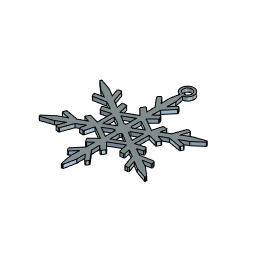
Snowflake 3 (Autodesk Fusion 360 design; units mm, degrees)
Autodesk Fusion 360 part; units mm, degrees
note: some values were not read from the file. Chosen so that the rebuilt part matches the saved one: which bodies a step acts on.
sketch "Sketch1" plane through (0, 0, 0) normal (0, 0, 1) x (1, 0, 0)
  line L0 (4.1638, 67.6877) -> (3.0782, 8.4572)
  line L1 (3.0782, 8.4572) -> (0, 0)
  line L2 (0, 0) -> (-3.0782, 8.4572)
  line L3 (-3.0782, 8.4572) -> (-4.1638, 67.6877)
  line L4 (-4.1638, 67.6877) -> (-1.1108, 83.3937)
  line L5 (-0.62, 83.7983) -> (0.62, 83.7983)
  line L6 (1.1108, 83.3937) -> (4.1638, 67.6877)
  line L7 (0, 0) -> (0, 83.7983) construction
  arc A0 (-0.62, 83.7983) -> (-1.1108, 83.3937) centre (-0.62, 83.2983) ccw
  arc A1 (1.1108, 83.3937) -> (0.62, 83.7983) centre (0.62, 83.2983) ccw
  dimension "d355" = 40
  dimension "d356" = 0.5
  dimension "d357" = 0.5
  dimension "d358" = 9
  dimension "d359" = 2.1
  dimension "d360" = 22
  dimension "d361" = 16
  dimension "d362" = 1.24
  constraint coincident L1.end L2.start
  constraint horizontal L5
  constraint vertical L7
  constraint symmetric L4 L6 L7
  constraint symmetric L0 L3 L7
  constraint symmetric L1 L2 L7
  constraint coincident L5 L7.end
  constraint tangent L4 A0
  constraint tangent L5 A0
  constraint tangent L5 A1
  constraint tangent L6 A1
  measures "d355" angle of L1 L2
  measures "d356" radius of A0
  measures "d357" radius of A1
  measures "d358" distance of L0.end L1.end
  measures "d359" angle of L0 L3
  measures "d360" angle of L4 L6
  measures "d361" distance of L0.start L6.start
  measures "d362" distance of L5.start L5.end
extrude "Extrude1" add sketch "Sketch1" along normal blind 5 makes body 1
pattern_circular "C-Pattern1" count 6 over 360 about axis through (0, 0, 1.75) along (0, 0, 1) of bodies 1 makes body 2 at (-42.0339, 23.0835, 0) makes body 3 at (-41.0079, -24.8607, 0) makes body 4 at (1.0261, -47.9442, 0) makes body 5 at (42.0339, -23.0835, 0) makes body 6 at (41.0079, 24.8607, 0)
sketch "Sketch2" plane through (0, 0, 0) normal (0, 0, 1) x (1, 0, 0)
  line L0 (1.1108, 83.3937) -> (4.1638, 67.6877)
  line L1 (4.1638, 67.6877) -> (3.0782, 8.4572)
  line L2 (3.0782, 8.4572) -> (0, 0)
  line L3 (0, 0) -> (-3.0782, 8.4572)
  line L4 (-3.0782, 8.4572) -> (-4.1638, 67.6877)
  line L5 (-4.1638, 67.6877) -> (-1.1108, 83.3937)
  arc A0 (-0.62, 83.7983) -> (-1.1108, 83.3937) centre (-0.62, 83.2983) ccw
  line L6 (-0.62, 83.7983) -> (0.62, 83.7983)
  arc A1 (1.1108, 83.3937) -> (0.62, 83.7983) centre (0.62, 83.2983) ccw
  line L7 (72.7765, 40.7349) -> (60.7011, 30.2379)
  line L8 (60.7011, 30.2379) -> (8.8633, 1.5628)
  line L9 (8.8633, 1.5628) -> (0, 0)
  line L10 (0, 0) -> (5.7851, 6.8944)
  line L11 (5.7851, 6.8944) -> (56.5374, 37.4498)
  line L12 (56.5374, 37.4498) -> (71.6657, 42.6589)
  arc A2 (72.2615, 42.4361) -> (71.6657, 42.6589) centre (71.8285, 42.1861) ccw
  line L13 (72.2615, 42.4361) -> (72.8815, 41.3622)
  arc A3 (72.7765, 40.7349) -> (72.8815, 41.3622) centre (72.4485, 41.1122) ccw
  line L14 (3.0782, 8.4572) -> (3.9851, 6.9024)
  line L15 (3.9851, 6.9024) -> (5.7851, 6.8944)
  line L16 (3.9851, 6.9024) -> (0, 0) construction
  dimension "d367" = 1.8
  constraint coincident L1.end L2.start
  constraint coincident L10.end L11.start
  constraint coincident L2.end L3.start
  constraint symmetric L2 L10 L16
  measures "d367" distance of L1.end L14.end
extrude "Extrude2" add sketch "Sketch2" along normal up to surface (5 mm away) separate body contours L2 L10 L14 L15 makes body 7
pattern_circular "C-Pattern2" count 6 over 360 about axis through (0, 0, 1.75) along (0, 0, 1) of bodies 7 makes body 8 at (-1.0261, 2.8191, 1.6667) makes body 9 at (-2.9544, 0.5209, 1.6667) makes body 10 at (-1.9284, -2.2981, 1.6667) makes body 11 at (1.0261, -2.8191, 1.6667) makes body 12 at (2.9544, -0.5209, 1.6667)
combine "Combine1" operation add target body 1 tool bodies 7 6 12 5 11 4 10 3 9 8 2
sketch "Sketch3" plane through (0, 0, 0) normal (0, 0, 1) x (1, 0, 0)
  line L0 (3.9453, 55.7691) -> (10.9697, 63.7874)
  line L1 (12.5222, 63.7282) -> (14.4807, 61.1147)
  line L2 (14.444, 59.8693) -> (3.7895, 47.2704)
  line L3 (3.7895, 47.2704) -> (3.9453, 55.7691)
  line L4 (-3.9453, 55.7691) -> (-10.9697, 63.7874)
  line L5 (-12.5222, 63.7282) -> (-14.4807, 61.1147)
  line L6 (-14.444, 59.8693) -> (-3.7895, 47.2704)
  line L7 (-3.7895, 47.2704) -> (-3.9453, 55.7691)
  line L8 (3.5792, 35.7959) -> (9.2878, 40.9035)
  line L9 (10.8187, 40.6617) -> (13.094, 36.7562)
  line L10 (12.9224, 35.5313) -> (3.407, 26.4)
  line L11 (3.407, 26.4) -> (3.5792, 35.7959)
  line L12 (-3.5792, 35.7959) -> (-9.2878, 40.9035)
  line L13 (-10.8187, 40.6617) -> (-13.094, 36.7562)
  line L14 (-12.9224, 35.5313) -> (-3.407, 26.4)
  line L15 (-3.407, 26.4) -> (-3.5792, 35.7959)
  line L16 (1.1108, 83.3937) -> (4.1638, 67.6877)
  line L17 (4.1638, 67.6877) -> (3.0782, 8.4572)
  line L18 (3.0782, 8.4572) -> (3.9851, 6.9024)
  line L19 (3.9851, 6.9024) -> (5.7851, 6.8944)
  line L20 (5.7851, 6.8944) -> (56.5374, 37.4498)
  line L21 (56.5374, 37.4498) -> (71.6657, 42.6589)
  arc A0 (72.2615, 42.4361) -> (71.6657, 42.6589) centre (71.8285, 42.1861) ccw
  line L22 (72.2615, 42.4361) -> (72.8815, 41.3622)
  arc A1 (72.7765, 40.7349) -> (72.8815, 41.3622) centre (72.4485, 41.1122) ccw
  line L23 (72.7765, 40.7349) -> (60.7011, 30.2379)
  line L24 (60.7011, 30.2379) -> (8.8633, 1.5628)
  line L25 (8.8633, 1.5628) -> (7.9702, 0)
  line L26 (7.9702, 0) -> (8.8633, -1.5628)
  line L27 (8.8633, -1.5628) -> (60.7011, -30.2379)
  line L28 (60.7011, -30.2379) -> (72.7765, -40.7349)
  arc A2 (72.8815, -41.3622) -> (72.7765, -40.7349) centre (72.4485, -41.1122) ccw
  line L29 (72.8815, -41.3622) -> (72.2615, -42.4361)
  arc A3 (71.6657, -42.6589) -> (72.2615, -42.4361) centre (71.8285, -42.1861) ccw
  line L30 (71.6657, -42.6589) -> (56.5374, -37.4498)
  line L31 (56.5374, -37.4498) -> (5.7851, -6.8944)
  line L32 (5.7851, -6.8944) -> (3.9851, -6.9024)
  line L33 (3.9851, -6.9024) -> (3.0782, -8.4572)
  line L34 (3.0782, -8.4572) -> (4.1638, -67.6877)
  line L35 (4.1638, -67.6877) -> (1.1108, -83.3937)
  arc A4 (0.62, -83.7983) -> (1.1108, -83.3937) centre (0.62, -83.2983) ccw
  line L36 (0.62, -83.7983) -> (-0.62, -83.7983)
  arc A5 (-1.1108, -83.3937) -> (-0.62, -83.7983) centre (-0.62, -83.2983) ccw
  line L37 (-1.1108, -83.3937) -> (-4.1638, -67.6877)
  line L38 (-4.1638, -67.6877) -> (-3.0782, -8.4572)
  line L39 (-3.0782, -8.4572) -> (-3.9851, -6.9024)
  line L40 (-3.9851, -6.9024) -> (-5.7851, -6.8944)
  line L41 (-5.7851, -6.8944) -> (-56.5374, -37.4498)
  line L42 (-56.5374, -37.4498) -> (-71.6657, -42.6589)
  arc A6 (-72.2615, -42.4361) -> (-71.6657, -42.6589) centre (-71.8285, -42.1861) ccw
  line L43 (-72.2615, -42.4361) -> (-72.8815, -41.3622)
  arc A7 (-72.7765, -40.7349) -> (-72.8815, -41.3622) centre (-72.4485, -41.1122) ccw
  line L44 (-72.7765, -40.7349) -> (-60.7011, -30.2379)
  line L45 (-60.7011, -30.2379) -> (-8.8633, -1.5628)
  line L46 (-8.8633, -1.5628) -> (-7.9702, 0)
  line L47 (-7.9702, 0) -> (-8.8633, 1.5628)
  line L48 (-8.8633, 1.5628) -> (-60.7011, 30.2379)
  line L49 (-60.7011, 30.2379) -> (-72.7765, 40.7349)
  arc A8 (-72.8815, 41.3622) -> (-72.7765, 40.7349) centre (-72.4485, 41.1122) ccw
  line L50 (-72.8815, 41.3622) -> (-72.2615, 42.4361)
  arc A9 (-71.6657, 42.6589) -> (-72.2615, 42.4361) centre (-71.8285, 42.1861) ccw
  line L51 (-71.6657, 42.6589) -> (-56.5374, 37.4498)
  line L52 (-56.5374, 37.4498) -> (-5.7851, 6.8944)
  line L53 (-5.7851, 6.8944) -> (-3.9851, 6.9024)
  line L54 (-3.9851, 6.9024) -> (-3.0782, 8.4572)
  line L55 (-3.0782, 8.4572) -> (-4.1638, 67.6877)
  line L56 (-4.1638, 67.6877) -> (-1.1108, 83.3937)
  arc A10 (-0.62, 83.7983) -> (-1.1108, 83.3937) centre (-0.62, 83.2983) ccw
  line L57 (-0.62, 83.7983) -> (0.62, 83.7983)
  arc A11 (1.1108, 83.3937) -> (0.62, 83.7983) centre (0.62, 83.2983) ccw
  line L58 (0, 83.7983) -> (0, 0) construction
  arc A12 (12.5222, 63.7282) -> (10.9697, 63.7874) centre (11.7219, 63.1285) ccw
  arc A13 (14.444, 59.8693) -> (14.4807, 61.1147) centre (13.6804, 60.515) ccw
  arc A14 (-10.9697, 63.7874) -> (-12.5222, 63.7282) centre (-11.7219, 63.1285) ccw
  arc A15 (-14.4807, 61.1147) -> (-14.444, 59.8693) centre (-13.6804, 60.515) ccw
  arc A16 (-9.2878, 40.9035) -> (-10.8187, 40.6617) centre (-9.9546, 40.1583) ccw
  arc A17 (-13.094, 36.7562) -> (-12.9224, 35.5313) centre (-12.23, 36.2528) ccw
  arc A18 (10.8187, 40.6617) -> (9.2878, 40.9035) centre (9.9546, 40.1583) ccw
  arc A19 (12.9224, 35.5313) -> (13.094, 36.7562) centre (12.23, 36.2528) ccw
  dimension "d372" = 1
  dimension "d373" = 1
  dimension "d374" = 1
  dimension "d375" = 10.66
  dimension "d376" = 3.2659
  dimension "d377" = 16.5
  dimension "d378" = 38.8131
  dimension "d379" = 40.17
  dimension "d380" = 1
  dimension "d381" = 1
  dimension "d382" = 2
  dimension "d383" = 4.52
  dimension "d384" = 7.66
  dimension "d385" = 47.13
  dimension "d386" = 26.4
  constraint collinear L11 L17
  constraint collinear L15 L55
  constraint collinear L7 L55
  constraint collinear L3 L17
  constraint midpoint L57 L58.start
  constraint coincident L58.end origin
  constraint symmetric L0 L4 L58
  constraint tangent L0 A12
  constraint tangent L1 A12
  constraint tangent L1 A13
  constraint tangent L2 A13
  constraint equal A12 A13
  constraint coincident L0.start L17
  constraint tangent L5 A14
  constraint tangent L4 A14
  constraint tangent L5 A15
  constraint tangent L6 A15
  constraint symmetric L1 L5 L58
  constraint symmetric L2 L6 L58
  constraint coincident L8.start L17
  constraint coincident L12.start L55
  constraint tangent L13 A16
  constraint tangent L12 A16
  constraint tangent L13 A17
  constraint tangent L14 A17
  constraint equal A16 A17
  constraint tangent L8 A18
  constraint tangent L9 A18
  constraint equal A16 A18
  constraint tangent L9 A19
  constraint tangent L10 A19
  constraint equal A16 A19
  constraint symmetric L8 L12 L58
  constraint symmetric L9 L13 L58
  constraint symmetric L10 L14 L58
  measures "d372" radius of A12
  measures "d373" radius of A14
  measures "d374" radius of A15
  measures "d375" distance of L0.start L0.end
  measures "d376" distance of L1.start L1.end
  measures "d377" distance of L2.end L2.start
  measures "d378" vertical distance of L2.end L17.end
  measures "d379" angle of L0 L17
  measures "d380" angle of L0 L2
  measures "d381" radius of A16
  measures "d382" angle of L8 L10
  measures "d383" distance of L9.start L9.end
  measures "d384" distance of L8.start L8.end
  measures "d385" angle of L8 L17
  measures "d386" vertical distance of L58.end L10.end
extrude "Extrude3" add sketch "Sketch3" along normal up to surface (5 mm away) separate body contours L0 L1 L2 L3 L17 A12 A13 | L8 L9 L10 L11 L17 A18 A19 | L4 L5 L6 L7 L55 A14 A15 | L12 L13 L14 L15 L55 A16 A17 makes body 13 at (6.6362, 32.5757, 0) makes body 14 at (-6.6362, 32.5757, 0) makes body 15 at (10.8925, 55.6697, 1.6667) makes body 16 at (-10.8925, 55.6697, 1.6667)
pattern_circular "C-Pattern3" count 6 over 360 about axis through (0, 0, 1.75) along (0, 0, 1) of bodies 13 14 15 16 makes body 17 at (-24.8933, 22.035, 0) makes body 18 at (-31.5295, -10.5407, 0) makes body 19 at (-6.6362, -32.5757, 0) makes body 20 at (24.8933, -22.035, 0) makes body 21 at (31.5295, 10.5407, 0) makes body 22 at (-31.5295, 10.5407, 0) makes body 23 at (-24.8933, -22.035, 0) makes body 24 at (6.6362, -32.5757, 0) makes body 25 at (31.5295, -10.5407, 0) makes body 26 at (24.8933, 22.035, 0) makes body 27 at (-42.7651, 37.268, 1.6667) makes body 28 at (-53.6576, -18.4016, 1.6667) makes body 29 at (-10.8925, -55.6697, 1.6667) makes body 30 at (42.7651, -37.268, 1.6667) makes body 31 at (53.6576, 18.4016, 1.6667) makes body 32 at (-53.6576, 18.4016, 3.3333) makes body 33 at (-42.7651, -37.268, 1.6667) makes body 34 at (10.8925, -55.6697, 3.3333) makes body 35 at (53.6576, -18.4016, 1.6667) makes body 36 at (42.7651, 37.268, 1.6667)
combine "Combine2" operation add target body 1 tool bodies 15 16 14 13 36 26 31 21 25 20 23 18 22 32 27 17 28 33 19 24 34 29 30 35
sketch "Sketch4" plane through (0, 0, 0) normal (0, 0, 1) x (1, 0, 0)
  line L0 (4.1458, 27.109) -> (21.4042, 17.1449)
  line L1 (3.3114, 21.1822) -> (16.6886, 13.4588)
  line L2 (1.1108, 83.3937) -> (4.1638, 67.6877)
  line L3 (4.1638, 67.6877) -> (3.9453, 55.7691)
  line L4 (3.9453, 55.7691) -> (10.9697, 63.7874)
  arc A0 (12.5222, 63.7282) -> (10.9697, 63.7874) centre (11.7219, 63.1285) ccw
  line L5 (12.5222, 63.7282) -> (14.4807, 61.1147)
  arc A1 (14.444, 59.8693) -> (14.4807, 61.1147) centre (13.6804, 60.515) ccw
  line L6 (14.444, 59.8693) -> (3.7895, 47.2704)
  line L7 (3.7895, 47.2704) -> (3.5792, 35.7959)
  line L8 (3.5792, 35.7959) -> (9.2878, 40.9035)
  arc A2 (10.8187, 40.6617) -> (9.2878, 40.9035) centre (9.9546, 40.1583) ccw
  line L9 (10.8187, 40.6617) -> (13.094, 36.7562)
  arc A3 (12.9224, 35.5313) -> (13.094, 36.7562) centre (12.23, 36.2528) ccw
  line L10 (12.9224, 35.5313) -> (3.407, 26.4)
  line L11 (3.407, 26.4) -> (3.0782, 8.4572)
  line L12 (3.0782, 8.4572) -> (3.9851, 6.9024)
  line L13 (3.9851, 6.9024) -> (5.7851, 6.8944)
  line L14 (5.7851, 6.8944) -> (21.1596, 16.1506)
  line L15 (21.1596, 16.1506) -> (24.3098, 28.9567)
  arc A4 (25.2848, 29.7179) -> (24.3098, 28.9567) centre (25.2808, 28.7179) ccw
  line L16 (25.2848, 29.7179) -> (29.8047, 29.7001)
  arc A5 (30.7796, 28.4952) -> (29.8047, 29.7001) centre (29.8008, 28.7001) ccw
  line L17 (30.7796, 28.4952) -> (29.2105, 20.9977)
  line L18 (29.2105, 20.9977) -> (39.0426, 26.917)
  line L19 (39.0426, 26.917) -> (44.6263, 42.4435)
  arc A6 (45.6866, 43.098) -> (44.6263, 42.4435) centre (45.5673, 42.1051) ccw
  line L20 (45.6866, 43.098) -> (48.9291, 42.7086)
  arc A7 (49.7567, 41.3938) -> (48.9291, 42.7086) centre (48.8099, 41.7157) ccw
  line L21 (49.7567, 41.3938) -> (46.3248, 31.3013)
  line L22 (46.3248, 31.3013) -> (56.5374, 37.4498)
  line L23 (56.5374, 37.4498) -> (71.6657, 42.6589)
  arc A8 (72.2615, 42.4361) -> (71.6657, 42.6589) centre (71.8285, 42.1861) ccw
  line L24 (72.2615, 42.4361) -> (72.8815, 41.3622)
  arc A9 (72.7765, 40.7349) -> (72.8815, 41.3622) centre (72.4485, 41.1122) ccw
  line L25 (72.7765, 40.7349) -> (60.7011, 30.2379)
  line L26 (60.7011, 30.2379) -> (50.2701, 24.4678)
  line L27 (50.2701, 24.4678) -> (60.7264, 22.3936)
  arc A10 (61.4513, 21.0196) -> (60.7264, 22.3936) centre (60.5318, 21.4128) ccw
  line L28 (61.4513, 21.0196) -> (60.1672, 18.0167)
  arc A11 (59.0703, 17.4258) -> (60.1672, 18.0167) centre (59.2478, 18.4099) ccw
  line L29 (59.0703, 17.4258) -> (42.8321, 20.3533)
  line L30 (42.8321, 20.3533) -> (32.7898, 14.7982)
  line L31 (32.7898, 14.7982) -> (40.0674, 12.4083)
  arc A12 (40.6234, 10.9616) -> (40.0674, 12.4083) centre (39.7554, 11.4582) ccw
  line L32 (40.6234, 10.9616) -> (38.3788, 7.0383)
  arc A13 (37.2322, 6.5745) -> (38.3788, 7.0383) centre (37.5108, 7.5349) ccw
  line L33 (37.2322, 6.5745) -> (24.5666, 10.2494)
  line L34 (24.5666, 10.2494) -> (8.8633, 1.5628)
  line L35 (8.8633, 1.5628) -> (7.9702, 0)
  line L36 (7.9702, 0) -> (8.8633, -1.5628)
  line L37 (8.8633, -1.5628) -> (24.5666, -10.2494)
  line L38 (24.5666, -10.2494) -> (37.2322, -6.5745)
  arc A14 (38.3788, -7.0383) -> (37.2322, -6.5745) centre (37.5108, -7.5349) ccw
  line L39 (38.3788, -7.0383) -> (40.6234, -10.9616)
  arc A15 (40.0674, -12.4083) -> (40.6234, -10.9616) centre (39.7554, -11.4582) ccw
  line L40 (40.0674, -12.4083) -> (32.7898, -14.7982)
  line L41 (32.7898, -14.7982) -> (42.8321, -20.3533)
  line L42 (42.8321, -20.3533) -> (59.0703, -17.4258)
  arc A16 (60.1672, -18.0167) -> (59.0703, -17.4258) centre (59.2478, -18.4099) ccw
  line L43 (60.1672, -18.0167) -> (61.4513, -21.0196)
  arc A17 (60.7264, -22.3936) -> (61.4513, -21.0196) centre (60.5318, -21.4128) ccw
  line L44 (60.7264, -22.3936) -> (50.2701, -24.4678)
  line L45 (50.2701, -24.4678) -> (60.7011, -30.2379)
  line L46 (60.7011, -30.2379) -> (72.7765, -40.7349)
  arc A18 (72.8815, -41.3622) -> (72.7765, -40.7349) centre (72.4485, -41.1122) ccw
  line L47 (72.8815, -41.3622) -> (72.2615, -42.4361)
  arc A19 (71.6657, -42.6589) -> (72.2615, -42.4361) centre (71.8285, -42.1861) ccw
  line L48 (71.6657, -42.6589) -> (56.5374, -37.4498)
  line L49 (56.5374, -37.4498) -> (46.3248, -31.3013)
  line L50 (46.3248, -31.3013) -> (49.7567, -41.3938)
  arc A20 (48.9291, -42.7086) -> (49.7567, -41.3938) centre (48.8099, -41.7157) ccw
  line L51 (48.9291, -42.7086) -> (45.6866, -43.098)
  arc A21 (44.6263, -42.4435) -> (45.6866, -43.098) centre (45.5673, -42.1051) ccw
  line L52 (44.6263, -42.4435) -> (39.0426, -26.917)
  line L53 (39.0426, -26.917) -> (29.2105, -20.9977)
  line L54 (29.2105, -20.9977) -> (30.7796, -28.4952)
  arc A22 (29.8047, -29.7001) -> (30.7796, -28.4952) centre (29.8008, -28.7001) ccw
  line L55 (29.8047, -29.7001) -> (25.2848, -29.7179)
  arc A23 (24.3098, -28.9567) -> (25.2848, -29.7179) centre (25.2808, -28.7179) ccw
  line L56 (24.3098, -28.9567) -> (21.1596, -16.1506)
  line L57 (21.1596, -16.1506) -> (5.7851, -6.8944)
  line L58 (5.7851, -6.8944) -> (3.9851, -6.9024)
  line L59 (3.9851, -6.9024) -> (3.0782, -8.4572)
  line L60 (3.0782, -8.4572) -> (3.407, -26.4)
  line L61 (3.407, -26.4) -> (12.9224, -35.5313)
  arc A24 (13.094, -36.7562) -> (12.9224, -35.5313) centre (12.23, -36.2528) ccw
  line L62 (13.094, -36.7562) -> (10.8187, -40.6617)
  arc A25 (9.2878, -40.9035) -> (10.8187, -40.6617) centre (9.9546, -40.1583) ccw
  line L63 (9.2878, -40.9035) -> (3.5792, -35.7959)
  line L64 (3.5792, -35.7959) -> (3.7895, -47.2704)
  line L65 (3.7895, -47.2704) -> (14.444, -59.8693)
  arc A26 (14.4807, -61.1147) -> (14.444, -59.8693) centre (13.6804, -60.515) ccw
  line L66 (14.4807, -61.1147) -> (12.5222, -63.7282)
  arc A27 (10.9697, -63.7874) -> (12.5222, -63.7282) centre (11.7219, -63.1285) ccw
  line L67 (10.9697, -63.7874) -> (3.9453, -55.7691)
  line L68 (3.9453, -55.7691) -> (4.1638, -67.6877)
  line L69 (4.1638, -67.6877) -> (1.1108, -83.3937)
  arc A28 (0.62, -83.7983) -> (1.1108, -83.3937) centre (0.62, -83.2983) ccw
  line L70 (0.62, -83.7983) -> (-0.62, -83.7983)
  arc A29 (-1.1108, -83.3937) -> (-0.62, -83.7983) centre (-0.62, -83.2983) ccw
  line L71 (-1.1108, -83.3937) -> (-4.1638, -67.6877)
  line L72 (-4.1638, -67.6877) -> (-3.9453, -55.7691)
  line L73 (-3.9453, -55.7691) -> (-10.9697, -63.7874)
  arc A30 (-12.5222, -63.7282) -> (-10.9697, -63.7874) centre (-11.7219, -63.1285) ccw
  line L74 (-12.5222, -63.7282) -> (-14.4807, -61.1147)
  arc A31 (-14.444, -59.8693) -> (-14.4807, -61.1147) centre (-13.6804, -60.515) ccw
  line L75 (-14.444, -59.8693) -> (-3.7895, -47.2704)
  line L76 (-3.7895, -47.2704) -> (-3.5792, -35.7959)
  line L77 (-3.5792, -35.7959) -> (-9.2878, -40.9035)
  arc A32 (-10.8187, -40.6617) -> (-9.2878, -40.9035) centre (-9.9546, -40.1583) ccw
  line L78 (-10.8187, -40.6617) -> (-13.094, -36.7562)
  arc A33 (-12.9224, -35.5313) -> (-13.094, -36.7562) centre (-12.23, -36.2528) ccw
  line L79 (-12.9224, -35.5313) -> (-3.407, -26.4)
  line L80 (-3.407, -26.4) -> (-3.0782, -8.4572)
  line L81 (-3.0782, -8.4572) -> (-3.9851, -6.9024)
  line L82 (-3.9851, -6.9024) -> (-5.7851, -6.8944)
  line L83 (-5.7851, -6.8944) -> (-21.1596, -16.1506)
  line L84 (-21.1596, -16.1506) -> (-24.3098, -28.9567)
  arc A34 (-25.2848, -29.7179) -> (-24.3098, -28.9567) centre (-25.2808, -28.7179) ccw
  line L85 (-25.2848, -29.7179) -> (-29.8047, -29.7001)
  arc A35 (-30.7796, -28.4952) -> (-29.8047, -29.7001) centre (-29.8008, -28.7001) ccw
  line L86 (-30.7796, -28.4952) -> (-29.2105, -20.9977)
  line L87 (-29.2105, -20.9977) -> (-39.0426, -26.917)
  line L88 (-39.0426, -26.917) -> (-44.6263, -42.4435)
  arc A36 (-45.6866, -43.098) -> (-44.6263, -42.4435) centre (-45.5673, -42.1051) ccw
  line L89 (-45.6866, -43.098) -> (-48.9291, -42.7086)
  arc A37 (-49.7567, -41.3938) -> (-48.9291, -42.7086) centre (-48.8099, -41.7157) ccw
  line L90 (-49.7567, -41.3938) -> (-46.3248, -31.3013)
  line L91 (-46.3248, -31.3013) -> (-56.5374, -37.4498)
  line L92 (-56.5374, -37.4498) -> (-71.6657, -42.6589)
  arc A38 (-72.2615, -42.4361) -> (-71.6657, -42.6589) centre (-71.8285, -42.1861) ccw
  line L93 (-72.2615, -42.4361) -> (-72.8815, -41.3622)
  arc A39 (-72.7765, -40.7349) -> (-72.8815, -41.3622) centre (-72.4485, -41.1122) ccw
  line L94 (-72.7765, -40.7349) -> (-60.7011, -30.2379)
  line L95 (-60.7011, -30.2379) -> (-50.2701, -24.4678)
  line L96 (-50.2701, -24.4678) -> (-60.7264, -22.3936)
  arc A40 (-61.4513, -21.0196) -> (-60.7264, -22.3936) centre (-60.5318, -21.4128) ccw
  line L97 (-61.4513, -21.0196) -> (-60.1672, -18.0167)
  arc A41 (-59.0703, -17.4258) -> (-60.1672, -18.0167) centre (-59.2478, -18.4099) ccw
  line L98 (-59.0703, -17.4258) -> (-42.8321, -20.3533)
  line L99 (-42.8321, -20.3533) -> (-32.7898, -14.7982)
  line L100 (-32.7898, -14.7982) -> (-40.0674, -12.4083)
  arc A42 (-40.6234, -10.9616) -> (-40.0674, -12.4083) centre (-39.7554, -11.4582) ccw
  line L101 (-40.6234, -10.9616) -> (-38.3788, -7.0383)
  arc A43 (-37.2322, -6.5745) -> (-38.3788, -7.0383) centre (-37.5108, -7.5349) ccw
  line L102 (-37.2322, -6.5745) -> (-24.5666, -10.2494)
  line L103 (-24.5666, -10.2494) -> (-8.8633, -1.5628)
  line L104 (-8.8633, -1.5628) -> (-7.9702, 0)
  line L105 (-7.9702, 0) -> (-8.8633, 1.5628)
  line L106 (-8.8633, 1.5628) -> (-24.5666, 10.2494)
  line L107 (-24.5666, 10.2494) -> (-37.2322, 6.5745)
  arc A44 (-38.3788, 7.0383) -> (-37.2322, 6.5745) centre (-37.5108, 7.5349) ccw
  line L108 (-38.3788, 7.0383) -> (-40.6234, 10.9616)
  arc A45 (-40.0674, 12.4083) -> (-40.6234, 10.9616) centre (-39.7554, 11.4582) ccw
  line L109 (-40.0674, 12.4083) -> (-32.7898, 14.7982)
  line L110 (-32.7898, 14.7982) -> (-42.8321, 20.3533)
  line L111 (-42.8321, 20.3533) -> (-59.0703, 17.4258)
  arc A46 (-60.1672, 18.0167) -> (-59.0703, 17.4258) centre (-59.2478, 18.4099) ccw
  line L112 (-60.1672, 18.0167) -> (-61.4513, 21.0196)
  arc A47 (-60.7264, 22.3936) -> (-61.4513, 21.0196) centre (-60.5318, 21.4128) ccw
  line L113 (-60.7264, 22.3936) -> (-50.2701, 24.4678)
  line L114 (-50.2701, 24.4678) -> (-60.7011, 30.2379)
  line L115 (-60.7011, 30.2379) -> (-72.7765, 40.7349)
  arc A48 (-72.8815, 41.3622) -> (-72.7765, 40.7349) centre (-72.4485, 41.1122) ccw
  line L116 (-72.8815, 41.3622) -> (-72.2615, 42.4361)
  arc A49 (-71.6657, 42.6589) -> (-72.2615, 42.4361) centre (-71.8285, 42.1861) ccw
  line L117 (-71.6657, 42.6589) -> (-56.5374, 37.4498)
  line L118 (-56.5374, 37.4498) -> (-46.3248, 31.3013)
  line L119 (-46.3248, 31.3013) -> (-49.7567, 41.3938)
  arc A50 (-48.9291, 42.7086) -> (-49.7567, 41.3938) centre (-48.8099, 41.7157) ccw
  line L120 (-48.9291, 42.7086) -> (-45.6866, 43.098)
  arc A51 (-44.6263, 42.4435) -> (-45.6866, 43.098) centre (-45.5673, 42.1051) ccw
  line L121 (-44.6263, 42.4435) -> (-39.0426, 26.917)
  line L122 (-39.0426, 26.917) -> (-29.2105, 20.9977)
  line L123 (-29.2105, 20.9977) -> (-30.7796, 28.4952)
  arc A52 (-29.8047, 29.7001) -> (-30.7796, 28.4952) centre (-29.8008, 28.7001) ccw
  line L124 (-29.8047, 29.7001) -> (-25.2848, 29.7179)
  arc A53 (-24.3098, 28.9567) -> (-25.2848, 29.7179) centre (-25.2808, 28.7179) ccw
  line L125 (-24.3098, 28.9567) -> (-21.1596, 16.1506)
  line L126 (-21.1596, 16.1506) -> (-5.7851, 6.8944)
  line L127 (-5.7851, 6.8944) -> (-3.9851, 6.9024)
  line L128 (-3.9851, 6.9024) -> (-3.0782, 8.4572)
  line L129 (-3.0782, 8.4572) -> (-3.407, 26.4)
  line L130 (-3.407, 26.4) -> (-12.9224, 35.5313)
  arc A54 (-13.094, 36.7562) -> (-12.9224, 35.5313) centre (-12.23, 36.2528) ccw
  line L131 (-13.094, 36.7562) -> (-10.8187, 40.6617)
  arc A55 (-9.2878, 40.9035) -> (-10.8187, 40.6617) centre (-9.9546, 40.1583) ccw
  line L132 (-9.2878, 40.9035) -> (-3.5792, 35.7959)
  line L133 (-3.5792, 35.7959) -> (-3.7895, 47.2704)
  line L134 (-3.7895, 47.2704) -> (-14.444, 59.8693)
  arc A56 (-14.4807, 61.1147) -> (-14.444, 59.8693) centre (-13.6804, 60.515) ccw
  line L135 (-14.4807, 61.1147) -> (-12.5222, 63.7282)
  arc A57 (-10.9697, 63.7874) -> (-12.5222, 63.7282) centre (-11.7219, 63.1285) ccw
  line L136 (-10.9697, 63.7874) -> (-3.9453, 55.7691)
  line L137 (-3.9453, 55.7691) -> (-4.1638, 67.6877)
  line L138 (-4.1638, 67.6877) -> (-1.1108, 83.3937)
  arc A58 (-0.62, 83.7983) -> (-1.1108, 83.3937) centre (-0.62, 83.2983) ccw
  line L139 (-0.62, 83.7983) -> (0.62, 83.7983)
  arc A59 (1.1108, 83.3937) -> (0.62, 83.7983) centre (0.62, 83.2983) ccw
  line L140 (0, 0) -> (10, 17.3205) construction
  dimension "d391" = 5.55
  dimension "d392" = 20
  constraint coincident L0.end L15
  constraint coincident L1.end L14
  constraint coincident L1.start L11
  constraint coincident L0.start L10
  constraint parallel L0 L1
  constraint coincident L140.start origin
  constraint midpoint L1 L140.end
  constraint perpendicular L1 L140
  measures "d391" distance of L0 L1
  measures "d392" distance of L140.start L140.end
extrude "Extrude4" add sketch "Sketch4" along normal up to surface (5 mm away) separate body contours L0 L1 L10 L11 L14 L15 makes body 37
pattern_circular "C-Pattern4" count 6 over 360 about axis through (0, 0, 1.75) along (0, 0, 1) of bodies 37 makes body 38 at (-14.0795, 19.2376, 0) makes body 39 at (-23.7, -2.5744, 0) makes body 40 at (-9.6205, -21.812, 0) makes body 41 at (14.0795, -19.2376, 0) makes body 42 at (23.7, 2.5744, 0)
combine "Combine3" operation add target body 1 tool bodies 37 38 39 40 41 42
sketch "Sketch5" plane through (0, 0, 0) normal (0, 0, 1) x (1, 0, 0)
  circle A0 centre (0, 87.7983) radius 6
  circle A1 centre (0, 87.7983) radius 9
  line L0 (-0.62, 83.7983) -> (0.62, 83.7983)
  line L1 (0, 83.7983) -> (0, 87.7983) construction
  dimension "d397" = 3
  dimension "d398" = 4
  dimension "d399" = 12
  constraint concentric A0 A1
  constraint midpoint L0 L1.start
  constraint coincident A0.centre A1.centre
  constraint vertical L1
  measures "d397" distance of A0 A1
  measures "d398" distance of L1.start A0.centre
  measures "d399" diameter of A0
extrude "Extrude5" add sketch "Sketch5" along normal up to surface (5 mm away) bodies 1
equation "d355 = 40 °"
equation "d359 = 2.1 °"
equation "d360 = 22 °"
equation "d379 = 40.17 °"
equation "d380 = 1 °"
equation "d382 = 2 °"
equation "d385 = 47.13 °"
